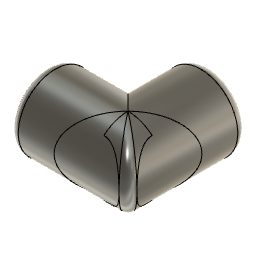
Connector_-_L_shaped (Autodesk Fusion 360 design; units mm, degrees)
Autodesk Fusion 360 part; units mm, degrees
cylinder "CylinderPrimitive1" add diameter 16.5 height 36.5 placed x (1, 0, 0) y (0, 1, 0) z (0, 0, 1) at (0, 0, 0) makes body 1
cylinder "CylinderPrimitive2" add diameter 16.5 height 36.5 placed x (1, 0, 0) y (0, 0, -1) z (0, 1, 0) at (30, 0, 0) separate body makes body 2
cylinder "CylinderPrimitive3" cut diameter 12.5 height -44 placed x (1, 0, 0) y (0, 0, 1) z (0, -1, 0) at (30, 0, 0) bodies 2
cylinder "CylinderPrimitive4" cut diameter 12.5 height 44 placed x (1, 0, 0) y (0, 1, 0) z (0, 0, 1) at (0, 0, 0) bodies 1
move_body "Move1" bodies 2 to x (1, 0, 0) y (0, 1, 0) z (0, 0, 1) at (-30, -18.25, 18.25)
combine "Combine1" operation add target body 1 tool bodies 2
cylinder "CylinderPrimitive5" cut diameter 12.5 height -44 placed x (1, 0, 0) y (0, 1, 0) z (0, 0, 1) at (0, 0, 36.5) bodies 1
cylinder "CylinderPrimitive6" cut diameter 12.5 height -44 placed x (1, 0, 0) y (0, 0, -1) z (0, 1, 0) at (0, 18.25, 18.25) bodies 1
fillet "Fillet1" radius 2 4 edges at (-7.6917, -2.9833, 36.5) (-7.6917, 18.25, 21.2333) (-7.6917, -18.25, 15.2667) (-7.6917, 2.9833, 0) on bodies 1
move_body "Move2" bodies 1 to x (0, 0, -1) y (0, 1, 0) z (1, 0, 0) at (-8.25, 0, -8.25)
move_body "Move3" bodies 1 to x (1, 0, 0) y (0, 1, 0) z (0, 0, 1) at (-10, 0, 0)
move_body "Move4" bodies 1 to x (1, 0, 0) y (0, 1, 0) z (0, 0, 1) at (0, 0, 16.5)
box "BoxPrimitive1" add length 50 width 30 height 22 placed x (0, -1, 0) y (1, 0, 0) z (0, 0, 1) at (-15, 25, 0) separate body makes body 3
move_body "Move5" bodies 3 to x (0.707107, -0.707107, 0) y (0.707107, 0.707107, 0) z (0, 0, 1) at (11.8701, -9.3431, 0)
combine "Combine2" operation cut target body 1 tool bodies 3
cylinder "CylinderPrimitive7" add diameter 16.5 height 16.5 placed x (1, 0, 0) y (0, 1, 0) z (0, 0, 1) at (25, 5, 0) separate body makes body 4
cylinder "CylinderPrimitive8" cut diameter 12.5 height -17 placed x (1, 0, 0) y (0, 1, 0) z (0, 0, 1) at (25, 5, 16.5) bodies 4
box "BoxPrimitive2" cut length 26 width 8.25 height 17 placed x (0, 1, 0) y (-1, 0, 0) z (0, 0, 1) at (25, -5, 0) bodies 4
copy_body "CopyPasteBodies1" bodies 4 makes body 5
move_body "Move6" bodies 5 to x (1, 0, 0) y (0, 1, 0) z (0, 0, 1) at (0, 11, 0)
move_body "Move7" bodies 4 to x (1, 0, 0) y (0, 0, 1) z (0, -1, 0) at (0, -3.25, 3.25)
move_body "Move8" bodies 4 to x (1, 0, 0) y (0, 1, 0) z (0, 0, 1) at (-25, 11.5, 0)
move_body "Move9" bodies 5 to x (0, -1, 0) y (0, 0, 1) z (-1, 0, 0) at (8.25, 24.75, -7.75)
move_body "Move10" bodies 5 to x (1, 0, 0) y (0, 1, 0) z (0, 0, 1) at (0, 0.25, 0)
combine "Combine3" operation add target body 1 tool bodies 4 5
cylinder "CylinderPrimitive9" add diameter 30 height 22 placed x (1, 0, 0) y (0, 1, 0) z (0, 0, 1) at (35, 0, 0) separate body makes body 6
cylinder "CylinderPrimitive10" cut diameter 16.5 height -22 placed x (1, 0, 0) y (0, 1, 0) z (0, 0, 1) at (35, 0, 22) bodies 6
box "BoxPrimitive3" cut length 35 width 18 height 22 placed x (0, -1, 0) y (1, 0, 0) z (0, 0, 1) at (35, 17, 0) bodies 6
copy_body "CopyPasteBodies2" bodies 6 makes body 7
move_body "Move11" bodies 7 to x (1, 0, 0) y (0, 1, 0) z (0, 0, 1) at (22, 0, 0)
move_body "Move12" bodies 7 to x (-1, 0, 0) y (0, 0, 1) z (0, 1, 0) at (57, -15, 8.25)
combine "Combine4" operation cut target body 1 tool bodies 7
move_body "Move13" bodies 6 to x (0, 1, 0) y (0, 0, 1) z (1, 0, 0) at (-10, -35, 8.25)
combine "Combine5" operation cut target body 1 tool bodies 6
fillet "Fillet2" radius 2 1 edges at (8.25, -8.25, 8.25) on bodies 1
